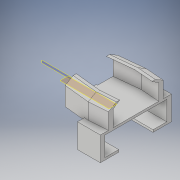
# Autodesk Inventor part: ESCFixation
Saved by Autodesk Inventor 2019 (Build 230136000, 136)
## iProperties
Created: 2018-09-20
Part Number: ESCFixation
Material: Generico
Document SubType Name: Modeling
Designer: acorbeau
Density: 1 g/cm^3
Appearance: Default
Author: acorbeau
Autodesk Inventor part; units mm, degrees
ref_plane "YZ Plane" through (0, 0, 0) normal (1, 0, 0) x (0, 1, 0)
ref_plane "XZ Plane" through (0, 0, 0) normal (0, 1, 0) x (-1, 0, 0)
ref_plane "XY Plane" through (0, 0, 0) normal (0, 0, 1) x (1, 0, 0)
sketch "Esquisse3" plane through (0, 0, 0) normal (0, 1, 0) x (-1, 0, 0)
  line L0 (0, 0) -> (11.196, -1.161)
  line L1 (11.196, -1.161) -> (11.196, -3.161)
  line L2 (11.196, -3.161) -> (0, -2)
  line L3 (0, -2) -> (-8.226, -2.628)
  line L4 (-8.226, -2.628) -> (-8.226, -0.628)
  line L5 (-8.226, -0.628) -> (0, 0)
  line L6 (0, 0) -> (0, -2) construction
  dimension "d10" = 0.628
  dimension "d11" = 1.161
  dimension "d12" = 11.256
  dimension "d13" = 8.226
  dimension "d14" = 2
  constraints: 14 end point, 3 parallel, 2 vertical
  measures "d10" vertical distance of L0.start L4.end
  measures "d11" vertical distance of L0.start L0.end
  measures "d12" distance of L0.start L0.end
  measures "d13" horizontal distance of L0.start L4.end
  measures "d14" distance of L0.end L1.end
extrude "Extrusion1" add sketch "Esquisse3" along normal blind 8
ref_plane "Plan de construction1" through (0, 10, 0) normal (0, 1, 0) x (1, 0, 0)
sketch "Esquisse4" plane through (0, 10, 0) normal (0, 1, 0) x (1, 0, 0)
  line L0 (8.226, 0.628) -> (8.226, 2.628) construction
  line L1 (8.226, 2.628) -> (0, 2) construction
  line L2 (8.226, 2.628) -> (0, 2) construction
  line L3 (0, 2) -> (-11.196, 3.161) construction
  line L4 (0, 2) -> (-11.196, 3.161) construction
  line L5 (-11.196, 3.161) -> (-11.196, 4.661) construction
  line L6 (-11.196, 4.661) -> (0, 3.5)
  line L7 (0, 3.5) -> (8.226, 4.128)
  line L8 (8.226, 2.628) -> (8.226, 4.128) construction
  line L9 (0, 2) -> (0, 3.5) construction
  line L10 (-11.196, 4.661) -> (-11.196, 6.0463)
  line L11 (-11.196, 6.0463) -> (-0.0003, 4.8853)
  line L12 (-0.0003, 4.8853) -> (8.226, 5.5133)
  line L13 (8.226, 5.5133) -> (8.226, 4.128)
  point P0 (0, 0)
  dimension "d18" = 1.5
  dimension "d19" = 1.5
  dimension "d20" = 1.5
  constraints: 22 end point, 4 vertical, 3 parallel, 2 collinear, 1 point on line
  measures "d18" distance of L7.end L0.end
  measures "d19" distance of L6.end L1.end
  measures "d20" distance of L5.end L3.end
loft "Lissage1" add profiles "Esquisse4" section 1 edges at (-5.598, 8, -0.5805) (4.113, 8, -0.314) (8.226, 8, -1.628) (4.113, 8, -2.314) (-5.598, 8, -2.5805) (-11.196, 8, -2.161)
sketch "Esquisse9" plane through (0, 0, 0) normal (0, -1, 0) x (1, 0, 0)
  line L0 (8.226, -0.628) -> (0, 0) projected
  line L1 (8.226, -0.628) -> (0, 0)
  line L2 (0, 0) -> (-11.196, -1.161) projected
  line L3 (0, 0) -> (-11.196, -1.161)
  line L4 (-11.196, -1.161) -> (-11.196, -22.84)
  line L5 (-11.196, -22.84) -> (0, -24)
  line L6 (0, -24) -> (8.226, -23.371)
  line L7 (8.226, -0.628) -> (8.226, -2.628) projected
  line L8 (8.226, -23.371) -> (8.226, -0.628)
  line L9 (0, 0) -> (0, -24) construction
  dimension "d29" = 24
  dimension "d30" = 22.743
  dimension "d31" = 21.679
  constraints: 14 end point, 3 collinear, 2 vertical
  measures "d29" distance of L0.end L5.end
  measures "d30" distance of L6.end L0.start
  measures "d31" distance of L2.end L4.end
extrude "Extrusion2" add sketch "Esquisse9" against normal blind 1
sketch "Esquisse10" plane through (0, 0, 0) normal (0, -1, 0) x (1, 0, 0)
  line L0 (8.226, -15.371) -> (-11.774, -15.371)
  line L1 (-11.774, -15.371) -> (-11.774, -8.628)
  line L2 (-11.774, -8.628) -> (8.226, -8.628)
  line L3 (8.226, -8.628) -> (8.226, -15.371)
  point P0 (8.226, -23.371)
  point P1 (8.226, -0.628)
  dimension "d34" = 8
  dimension "d35" = 8
  dimension "d36" = 20
  constraints: 8 end point, 2 parallel, 1 horizontal, 1 perpendicular, 1 point on line
  measures "d34" distance of point (8.226, -23.371) L0.start
  measures "d35" distance of point (8.226, -0.628) L2.end
  measures "d36" distance of L0.start L0.end
extrude "Extrusion3" add sketch "Esquisse10" against normal blind 1
ref_plane "Plan de construction3" through (-11.196, 0, -12.5995) normal (0, 0, -1) x (-1, 0, 0)
mirror "Symétrie2" about plane through (-11.196, 0, -12.5995) normal (0, 0, -1) of "Extrusion1", "Lissage1"
sketch "Esquisse11" plane through (0, 0, 0) normal (0, -1, 0) x (1, 0, 0)
  line L0 (8.226, -28.0995) -> (-1.774, -28.0995)
  line L1 (-1.774, -28.0995) -> (-1.774, 2.9005)
  line L2 (-1.774, 2.9005) -> (8.226, 2.9005)
  line L3 (8.226, 2.9005) -> (8.226, -28.0995) construction
  line L4 (8.226, -28.0995) -> (8.226, -24.571)
  line L5 (8.226, -24.571) -> (8.226, -0.628) projected
  line L6 (8.226, -0.628) -> (8.226, 2.9005)
  point P0 (0, 0)
  dimension "d40" = 31
  dimension "d41" = 10
  constraints: 12 end point, 3 collinear, 2 parallel, 1 horizontal, 1 perpendicular, 1 point on line
  measures "d40" distance of L2.end L0.start
  measures "d41" distance of L0.start L0.end
extrude "Extrusion4" add sketch "Esquisse11" against normal blind 1
sketch "Esquisse12" plane through (0, 0, 0) normal (0, -1, 0) x (1, 0, 0)
  line L0 (8.226, -28.0995) -> (-1.774, -28.0995) projected
  line L1 (8.226, -28.0995) -> (-1.774, -28.0995)
  line L2 (-1.774, -28.0995) -> (-1.774, -26.0995)
  line L3 (-1.774, -28.0995) -> (-1.774, -25.015) construction
  line L4 (8.226, -24.571) -> (8.226, -28.0995) construction
  line L5 (8.226, -26.0995) -> (-1.774, -26.0995)
  line L6 (8.226, -28.0995) -> (8.226, -26.0995)
  point P0 (0, 0)
  dimension "d44" = 2
  constraints: 8 end point, 2 perpendicular, 2 point on line, 1 collinear
  measures "d44" distance of L0.end L2.end
extrude "Extrusion5" add sketch "Esquisse12" along normal blind 8.5
mirror "Symétrie3" about plane through (-11.196, 0, -12.5995) normal (0, 0, -1) of "Extrusion5"
sketch "Esquisse13" plane through (0, -8.5, 0) normal (0, -1, 0) x (1, 0, 0)
  line L0 (8.226, -24.571) -> (8.226, -28.0995) projected
  line L1 (-1.774, 2.9005) -> (8.226, 2.9005) projected
  line L2 (8.226, -28.0995) -> (-1.774, -28.0995)
  line L3 (-1.774, -28.0995) -> (-1.774, 2.9005)
  line L4 (-1.774, 2.9005) -> (8.226, 2.9005)
  line L5 (8.226, 2.9005) -> (8.226, -28.0995)
  point P0 (0, 0)
  constraints: 8 end point, 2 parallel, 1 horizontal, 1 perpendicular
extrude "Extrusion6" add sketch "Esquisse13" along normal blind 1
sketch "Esquisse14" plane through (0, -9.5, 0) normal (0, -1, 0) x (1, 0, 0)
  line L0 (-1.774, -26.0995) -> (-1.774, 0.9005) construction
  line L1 (8.226, 0.9005) -> (8.226, -26.0995) construction
  line L2 (-1.774, -20.0995) -> (8.226, -20.0995)
  line L3 (8.226, -20.0995) -> (8.226, -5.0995)
  line L4 (8.226, -5.0995) -> (-1.774, -5.0995)
  line L5 (-1.774, -5.0995) -> (-1.774, -20.0995)
  line L6 (-1.774, -28.0995) -> (8.226, -28.0995) construction
  line L7 (8.226, 2.9005) -> (-1.774, 2.9005) construction
  line L8 (-1.774, -20.0995) -> (-1.774, -5.0995)
  line L9 (8.226, -5.0995) -> (8.226, -20.0995)
  point P0 (0, 0)
  dimension "d49" = 8
  dimension "d50" = 8
  constraints: 12 end point, 3 parallel, 2 point on line, 1 collinear, 1 horizontal, 1 perpendicular
  measures "d49" distance between parallel lines of L6 L2
  measures "d50" distance between parallel lines of L7 L4
extrude "Extrusion7" cut sketch "Esquisse14" against normal blind 1
